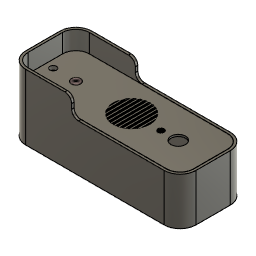
voipdoorbell-modeled (Autodesk Fusion 360 design; units mm, degrees)
Autodesk Fusion 360 part; units mm, degrees
sketch "Sketch1" plane through (0, 0, 0) normal (0, 1, 0) x (1, 0, 0)
  line L0 (-29, 11.5) -> (29, 11.5) construction
  line L1 (29, 11.5) -> (29, -11.5) construction
  line L2 (29, -11.5) -> (-29, -11.5) construction
  line L3 (-29, -11.5) -> (-29, 11.5) construction
  line L4 (-29, 11.5) -> (29, -11.5) construction
  line L5 (29, 11.5) -> (-29, -11.5) construction
  circle A0 centre (-29, 11.5) radius 1.25
  circle A1 centre (29, 11.5) radius 1.25
  circle A2 centre (29, -11.5) radius 1.25
  circle A3 centre (-29, -11.5) radius 1.25
  circle A4 centre (-29, 11.5) radius 2.75
  circle A5 centre (29, 11.5) radius 2.75
  circle A6 centre (29, -11.5) radius 2.75
  circle A7 centre (-29, -11.5) radius 2.75
  line L6 (56.5, 25) -> (-56.5, 25)
  line L7 (-67.5, 14) -> (-67.5, -14)
  line L8 (-56.5, -25) -> (56.5, -25)
  line L9 (67.5, -14) -> (67.5, 14)
  line L10 (67.5, 25) -> (-67.5, -25) construction
  line L11 (-67.5, 25) -> (67.5, -25) construction
  arc A8 (-67.5, -14) -> (-56.5, -25) centre (-56.5, -14) ccw
  arc A9 (-56.5, 25) -> (-67.5, 14) centre (-56.5, 14) ccw
  arc A10 (67.5, 14) -> (56.5, 25) centre (56.5, 14) ccw
  arc A11 (56.5, -25) -> (67.5, -14) centre (56.5, -14) ccw
  line L12 (69.5, -14) -> (69.5, 14)
  arc A12 (69.5, 14) -> (56.5, 27) centre (56.5, 14) ccw
  line L13 (56.5, 27) -> (-56.5, 27)
  arc A13 (-56.5, 27) -> (-69.5, 14) centre (-56.5, 14) ccw
  line L14 (-69.5, 14) -> (-69.5, -14)
  arc A14 (-69.5, -14) -> (-56.5, -27) centre (-56.5, -14) ccw
  line L15 (-56.5, -27) -> (56.5, -27)
  arc A15 (56.5, -27) -> (69.5, -14) centre (56.5, -14) ccw
  circle A16 centre (60, 0) radius 5
  circle A17 centre (56.5, -14) radius 1.5
  circle A18 centre (56.5, 14) radius 1.5
  circle A19 centre (-56.5, -14) radius 1.5
  circle A20 centre (-56.5, 14) radius 1.5
  dimension "d1" = 58
  dimension "d2" = 23
  dimension "d3" = 2.5
  dimension "d4" = 2.5
  dimension "d5" = 2.5
  dimension "d6" = 2.5
  dimension "d7" = 1.5
  dimension "d8" = 1.5
  dimension "d9" = 1.5
  dimension "d10" = 1.5
  dimension "d11" = 11
  dimension "d12" = 11
  dimension "d13" = 11
  dimension "d14" = 11
  dimension "d15" = 135
  dimension "d16" = 50
  dimension "d17" = 2
  dimension "d53" = 10
  dimension "d79" = 3
  dimension "d80" = 3
  dimension "d81" = 3
  dimension "d82" = 3
  constraint horizontal L0
  constraint perpendicular L0 L1
  constraint parallel L0 L2
  constraint parallel L1 L3
  constraint coincident L4 origin
  constraint coincident L5 origin
  constraint coincident L0.start L3.end
  constraint coincident L0.end L1.start
  constraint coincident L1.end L2.start
  constraint coincident L2.end L3.start
  constraint horizontal L6
  constraint perpendicular L6 L7
  constraint parallel L6 L8
  constraint parallel L7 L9
  constraint coincident L10 origin
  constraint coincident L11 origin
  constraint coincident L10.end L8
  constraint coincident L10.end L7
  constraint tangent L8 A8
  constraint tangent L7 A8
  constraint coincident L11.start L7
  constraint coincident L11.start L6
  constraint tangent L7 A9
  constraint tangent L6 A9
  constraint coincident L10.start L9
  constraint coincident L10.start L6
  constraint tangent L9 A10
  constraint tangent L6 A10
  constraint coincident L11.end L9
  constraint coincident L11.end L8
  constraint tangent L9 A11
  constraint tangent L8 A11
  constraint concentric A11 A17
  constraint concentric A10 A18
  constraint concentric A8 A19
  constraint concentric A9 A20
  measures "d1" distance of L0.start L0.end
  measures "d2" distance of L0.end L1.end
  measures "d3" diameter of A0
  measures "d4" diameter of A3
  measures "d5" diameter of A1
  measures "d6" diameter of A2
  measures "d11" radius of A8
  measures "d12" radius of A9
  measures "d13" radius of A10
  measures "d14" radius of A11
  measures "d15" distance of L7 L9
  measures "d16" distance of L6 L8
  measures "d53" diameter of A16
  measures "d79" diameter of A20
  measures "d80" diameter of A19
  measures "d81" diameter of A17
  measures "d82" diameter of A18
other "Base Mesh Feature1"
other "Base Mesh Feature2"
other "Modify1"
other "Modify2"
other "Modify3"
extrude "Extrude1" add sketch "Sketch1" against normal blind 2 contours A0 | A1 | A2 | A3 | A4 | A5 | A6 | A7 | L6 L7 L8 L9 A8 A9 A10 A11 | L12 A12 L13 A13 L14 A14 L15 A15 | A16 | A17 | A18 | A19 | A20 makes body 1
extrude "Extrude2" add sketch "Sketch1" along normal blind 2 contours A4 | A5 | A6 | A7 bodies 1
extrude "Extrude3" add sketch "Sketch1" along normal blind 35 contours L12 A12 L13 A13 L14 A14 L15 A15 bodies 1
sketch "Sketch2" plane through (0, 35, 0) normal (0, 1, 0) x (-1, 0, 0)
  arc A0 (-56.5, 25) -> (-67.5, 14) centre (-56.5, 14) ccw
  line L0 (-56.5, 25) -> (56.5, 25)
  arc A1 (67.5, 14) -> (56.5, 25) centre (56.5, 14) ccw
  line L1 (67.5, 14) -> (67.5, -14)
  arc A2 (56.5, -25) -> (67.5, -14) centre (56.5, -14) ccw
  line L2 (56.5, -25) -> (-56.5, -25)
  arc A3 (-67.5, -14) -> (-56.5, -25) centre (-56.5, -14) ccw
  line L3 (-67.5, -14) -> (-67.5, 14)
  arc A4 (-56.5, 27) -> (-69.5, 14) centre (-56.5, 14) ccw
  line L4 (-69.5, 14) -> (-69.5, -14)
  arc A5 (-69.5, -14) -> (-56.5, -27) centre (-56.5, -14) ccw
  line L5 (-56.5, -27) -> (56.5, -27)
  arc A6 (56.5, -27) -> (69.5, -14) centre (56.5, -14) ccw
  line L6 (69.5, -14) -> (69.5, 14)
  arc A7 (69.5, 14) -> (56.5, 27) centre (56.5, 14) ccw
  line L7 (56.5, 27) -> (-56.5, 27)
  line L8 (67.35, 14) -> (67.35, -14)
  arc A8 (56.5, -24.85) -> (67.35, -14) centre (56.5, -14) ccw
  line L9 (56.5, -24.85) -> (-56.5, -24.85)
  arc A9 (-67.35, -14) -> (-56.5, -24.85) centre (-56.5, -14) ccw
  line L10 (-67.35, -14) -> (-67.35, 14)
  arc A10 (-56.5, 24.85) -> (-67.35, 14) centre (-56.5, 14) ccw
  line L11 (-56.5, 24.85) -> (56.5, 24.85)
  arc A11 (67.35, 14) -> (56.5, 24.85) centre (56.5, 14) ccw
  circle A12 centre (42.5, 0) radius 3.75
  line L12 (54.25, 10.5) -> (42, 10.5) construction
  line L13 (42, 10.5) -> (42, -10.5) construction
  line L14 (42, -10.5) -> (54.25, -10.5) construction
  line L15 (54.25, -10.5) -> (54.25, 10.5) construction
  circle A13 centre (42, 10.5) radius 1
  circle A14 centre (42, -10.5) radius 1
  circle A15 centre (54.25, -10.5) radius 1
  circle A16 centre (54.25, 10.5) radius 1
  circle A17 centre (-41, 0) radius 6
  circle A18 centre (-27, 0) radius 2.5
  circle A19 centre (-3, 0) radius 15
  circle A20 centre (-3, 0) radius 18.5
  line L16 (-56.5, 23.3) -> (56.5, 23.3)
  arc A21 (65.8, 14) -> (56.5, 23.3) centre (56.5, 14) ccw
  line L17 (65.8, 14) -> (65.8, -14)
  arc A22 (56.5, -23.3) -> (65.8, -14) centre (56.5, -14) ccw
  line L18 (56.5, -23.3) -> (-56.5, -23.3)
  arc A23 (-65.8, -14) -> (-56.5, -23.3) centre (-56.5, -14) ccw
  line L19 (-65.8, -14) -> (-65.8, 14)
  arc A24 (-56.5, 23.3) -> (-65.8, 14) centre (-56.5, 14) ccw
  circle A25 centre (42, -10.5) radius 2
  circle A26 centre (54.25, -10.5) radius 2
  circle A27 centre (54.25, 10.5) radius 2
  circle A28 centre (42, 10.5) radius 2
  dimension "d24" = -0.15
  dimension "d25" = 7.5
  dimension "d26" = 25
  dimension "d27" = 25
  dimension "d28" = 2
  dimension "d29" = 2
  dimension "d30" = 2
  dimension "d31" = 2
  dimension "d32" = 21
  dimension "d33" = 12.25
  dimension "d34" = 10.5
  dimension "d35" = 0.5
  dimension "d37" = 12
  dimension "d39" = 30
  dimension "d40" = 37
  dimension "d41" = 5
  dimension "d42" = 1.7
  dimension "d126" = 4
  dimension "d127" = 4
  dimension "d128" = 4
  dimension "d129" = 4
  constraint horizontal L12
  constraint vertical L13
  constraint horizontal L14
  constraint vertical L15
  constraint coincident L12.end L13.start
  constraint coincident L13.end L14.start
  constraint coincident L14.end L15.start
  constraint coincident L12.start L15.end
  constraint concentric A19 A20
  constraint concentric A16 A27
  constraint concentric A13 A28
  measures "d25" diameter of A12
  measures "d26" distance of L1 A12.centre
  measures "d27" distance of L2 A12.centre
  measures "d28" diameter of A13
  measures "d29" diameter of A14
  measures "d30" diameter of A15
  measures "d31" diameter of A16
  measures "d32" distance of L12.end L13.end
  measures "d33" distance of L12.start L12.end
  measures "d34" distance of A12.centre L12
  measures "d35" distance of A12.centre L13
  measures "d37" diameter of A17
  measures "d39" diameter of A19
  measures "d40" diameter of A20
  measures "d41" diameter of A18
  measures "d126" diameter of A25
  measures "d127" diameter of A26
  measures "d128" diameter of A27
  measures "d129" diameter of A28
extrude "Extrude4" add sketch "Sketch2" against normal blind 24.95 separate body contours L8 A8 L9 A9 L10 A10 L11 A11 makes body 2
extrude "Extrude5" add sketch "Sketch2" along normal blind 1.5 contours L8 A8 L9 A9 L10 A10 L11 A11 | A13 | A14 | A15 | A16 | A20 | L16 A21 L17 A22 L18 A23 L19 A24 | A25 | A26 | A27 | A28 bodies 2
extrude "Extrude7" cut sketch "Sketch1" against normal blind 16 contours A16 bodies 1
extrude "Extrude8" add 1 faces at (18.8333, 35, 25.6667) along direction (0, 1, 0) blind 1.5 on bodies 1 bodies 1
sketch "Sketch4" plane through (0, 36.5, 0) normal (0, 1, 0) x (-1, 0, 0)
  arc A0 (-56.5, 25) -> (-67.5, 14) centre (-56.5, 14) ccw
  line L0 (-56.5, 25) -> (56.5, 25)
  arc A1 (67.5, 14) -> (56.5, 25) centre (56.5, 14) ccw
  line L1 (67.5, 14) -> (67.5, -14)
  arc A2 (56.5, -25) -> (67.5, -14) centre (56.5, -14) ccw
  line L2 (56.5, -25) -> (-56.5, -25)
  arc A3 (-67.5, -14) -> (-56.5, -25) centre (-56.5, -14) ccw
  line L3 (-67.5, -14) -> (-67.5, 14)
  arc A4 (-56.5, 27) -> (-69.5, 14) centre (-56.5, 14) ccw
  line L4 (-69.5, 14) -> (-69.5, -14)
  arc A5 (-69.5, -14) -> (-56.5, -27) centre (-56.5, -14) ccw
  line L5 (-56.5, -27) -> (56.5, -27)
  arc A6 (56.5, -27) -> (69.5, -14) centre (56.5, -14) ccw
  line L6 (69.5, -14) -> (69.5, 14)
  arc A7 (69.5, 14) -> (56.5, 27) centre (56.5, 14) ccw
  line L7 (56.5, 27) -> (-56.5, 27)
  line L8 (19, 39) -> (19, -40)
  constraint vertical L8
extrude "Extrude9" add sketch "Sketch4" along normal blind 15 contours L0 A1 L1 A2 L2 L5 A6 L6 A7 L7 L8 bodies 1
fillet "Fillet3" radius 5.5 2 edges at (-19, 51.5, -26) (-19, 51.5, 26) on bodies 1
fillet "Fillet4" radius 5.5 2 edges at (-19, 36.5, 26) (-19, 36.5, -26) on bodies 1
sketch "Sketch5" plane through (-67.35, 0, 0) normal (-1, 0, 0) x (0, 0, 1)
  line L0 (-14, 36.5) -> (-14, 10.05)
  line L1 (-14, 10.05) -> (14, 10.05)
  line L2 (14, 10.05) -> (14, 36.5)
  line L3 (14, 36.5) -> (-14, 36.5)
  line L4 (4.9486, 10.05) -> (-4.9486, 10.05)
  line L5 (-4.9486, 10.05) -> (-4.9486, 31.95)
  line L6 (-4.9486, 31.95) -> (4.9486, 31.95)
  line L7 (4.9486, 31.95) -> (4.9486, 10.05)
  line L8 (4.9486, 10.05) -> (-4.9486, 31.95) construction
  line L9 (-4.9486, 10.05) -> (4.9486, 31.95) construction
  point P0 (0, 21)
  constraint horizontal L4
  constraint perpendicular L4 L5
  constraint parallel L4 L6
  constraint parallel L5 L7
  constraint coincident L8 P0
  constraint coincident L9 P0
  constraint coincident L1 L4.start
extrude "Extrude10" cut sketch "Sketch5" against normal blind 5 contours L1 L4 L5 L6 L7 bodies 2
extrude "Extrude11" cut 1 faces at (-66.3167, 31.95, 1.6495) along direction (0, 1, 0) blind 3 on bodies 2 bodies 2
sketch "Sketch6" plane through (-67.5, 0, 0) normal (1, 0, 0) x (0, 0, -1)
  line L0 (-14, 0) -> (14, 0)
  line L1 (14, 0) -> (14, 51.5)
  line L2 (14, 51.5) -> (-14, 51.5)
  line L3 (-14, 51.5) -> (-14, 0)
  line L4 (4.2362, 7.1464) -> (-4.2553, 7.1464)
  line L5 (-4.2553, 7.1464) -> (-4.2553, 24.7678)
  line L6 (-4.2553, 24.7678) -> (4.2362, 24.7678)
  line L7 (4.2362, 24.7678) -> (4.2362, 7.1464)
  line L8 (4.2362, 7.1464) -> (-4.2553, 24.7678) construction
  line L9 (-4.2553, 7.1464) -> (4.2362, 24.7678) construction
  point P0 (-0.0095, 15.9571)
  constraint horizontal L4
  constraint perpendicular L4 L5
  constraint parallel L4 L6
  constraint parallel L5 L7
  constraint coincident L8 P0
  constraint coincident L9 P0
extrude "Extrude12" add sketch "Sketch6" along normal blind 4.5 separate body contours L4 L5 L6 L7 makes body 3
sketch "Sketch7" plane through (0, 7.1464, 0) normal (0, -1, 0) x (1, 0, 0)
  line L0 (-67.5, 4.2553) -> (-67.5, -4.2362)
  line L1 (-67.5, -4.2362) -> (-63, -4.2362)
  line L2 (-63, -4.2362) -> (-63, 4.2553)
  line L3 (-63, 4.2553) -> (-67.5, 4.2553)
  circle A0 centre (-49.4164, -0.0071) radius 1.25
  circle A1 centre (-49.4164, -0.0071) radius 1.5
  dimension "d70" = 2.5
  dimension "d132" = 3
  constraint concentric A0 A1
  measures "d70" diameter of A0
  measures "d132" diameter of A1
extrude "Extrude14" add 1 faces at (-63, 18.894, 1.4248) along direction (1, 0, 0) blind 0.5 on bodies 3 bodies 3
extrude "Extrude16" add 1 faces at (-67.5, 18.894, 1.4248) along direction (-1, 0, 0) blind 1 on bodies 3 bodies 3 1
extrude "Extrude17" cut sketch "Sketch1" against normal blind 11 contours A17 | A18 | A19 | A20 bodies 3
sketch "Sketch9" plane through (0, 36.5, 0) normal (0, 1, 0) x (-1, 0, 0)
  circle A0 centre (42.5, 0) radius 3.75
  circle A1 centre (-3, 0) radius 15
  circle A2 centre (-41, 0) radius 6
  circle A3 centre (-27, 0) radius 2.5
  arc A4 (56.5, -24.85) -> (67.35, -14) centre (56.5, -14) ccw
  line L0 (67.35, -14) -> (67.35, 14)
  arc A5 (67.35, 14) -> (56.5, 24.85) centre (56.5, 14) ccw
  line L1 (56.5, 24.85) -> (-56.5, 24.85)
  arc A6 (-56.5, 24.85) -> (-67.35, 14) centre (-56.5, 14) ccw
  line L2 (-67.35, 14) -> (-67.35, -14)
  arc A7 (-67.35, -14) -> (-56.5, -24.85) centre (-56.5, -14) ccw
  line L3 (-56.5, -24.85) -> (56.5, -24.85)
  line L4 (13, 20) -> (13, -20)
  line L5 (11.5, 20) -> (11.5, -20)
  line L6 (10, 20) -> (10, -20)
  line L7 (8.5, 20) -> (8.5, -20)
  line L8 (7, 20) -> (7, -20)
  line L9 (5.5, 20) -> (5.5, -20)
  line L10 (4, 20) -> (4, -20)
  line L11 (2.5, 20) -> (2.5, -20)
  line L12 (1, 20) -> (1, -20)
  line L13 (-0.5, 20) -> (-0.5, -20)
  line L14 (-2, 20) -> (-2, -20)
  line L15 (-3.5, 20) -> (-3.5, -20)
  line L16 (-5, 20) -> (-5, -20)
  line L17 (-6.5, 20) -> (-6.5, -20)
  line L18 (-8, 20) -> (-8, -20)
  line L19 (-9.5, 20) -> (-9.5, -20)
  line L20 (-11, 20) -> (-11, -20)
  line L21 (-12.5, 20) -> (-12.5, -20)
  line L22 (-14, 20) -> (-14, -20)
  line L23 (-15.5, 20) -> (-15.5, -20)
  line L24 (-17, 20) -> (-17, -20)
  line L25 (-18.5, 20) -> (-18.5, -20)
  line L26 (-24.757, 5.9816) -> (-24.757, -6.5184)
  line L27 (-25.257, 5.9816) -> (-25.257, -6.5184)
  line L28 (-25.757, 5.9816) -> (-25.757, -6.5184)
  line L29 (-26.257, 5.9816) -> (-26.257, -6.5184)
  line L30 (-26.757, 5.9816) -> (-26.757, -6.5184)
  line L31 (-27.257, 5.9816) -> (-27.257, -6.5184)
  line L32 (-27.757, 5.9816) -> (-27.757, -6.5184)
  line L33 (-28.257, 5.9816) -> (-28.257, -6.5184)
  line L34 (-28.757, 5.9816) -> (-28.757, -6.5184)
  line L35 (-29.257, 5.9816) -> (-29.257, -6.5184)
  line L36 (-29.757, 5.9816) -> (-29.757, -6.5184)
  dimension "d85" = 1.5
  dimension "d86" = 3
  dimension "d87" = 4.5
  dimension "d88" = 6
  dimension "d89" = 7.5
  dimension "d90" = 9
  dimension "d91" = 10.5
  dimension "d92" = 12
  dimension "d93" = 13.5
  dimension "d94" = 15
  dimension "d95" = 16.5
  dimension "d96" = 18
  dimension "d97" = 19.5
  dimension "d98" = 21
  dimension "d99" = 22.5
  dimension "d100" = 24
  dimension "d101" = 25.5
  dimension "d102" = 27
  dimension "d103" = 28.5
  dimension "d104" = 30
  dimension "d105" = 31.5
  dimension "d114" = 0.5
  dimension "d115" = 1
  dimension "d116" = 1.5
  dimension "d117" = 2
  dimension "d118" = 2.5
  dimension "d119" = 3
  dimension "d120" = 3.5
  dimension "d121" = 4
  dimension "d122" = 4.5
  dimension "d123" = 5
  constraint perpendicular L3 L4
  constraint vertical L26
extrude "Extrude18" add sketch "Sketch9" against normal blind 1.5 contours A1 L5 | A1 L5 L6 | A1 L6 L7 | A1 L7 L8 | A1 L8 L9 | A1 L9 L10 | A1 L10 L11 | A1 L11 L12 | A1 L12 L13 | A1 L13 L14 | A1 L14 L15 | A1 L15 L16 | A1 L16 L17 | A1 L17 L18 | A1 L18 L19 | A1 L19 L20 | A1 L20 L21 | A1 L21 L22 | A1 L22 L23 | A1 L23 L24 | A1 L24 bodies 2
extrude "Extrude19" cut sketch "Sketch9" against normal blind 5 contours A1 L5 L6 | A1 L7 L8 | A1 L9 L10 | A1 L11 L12 | A1 L13 L14 | A1 L15 L16 | A1 L17 L18 | A1 L19 L20 | A1 L21 L22 | A1 L23 L24 bodies 2
extrude "Extrude20" cut sketch "Sketch9" against normal blind 1 contours A1 L5 | A1 L6 L7 | A1 L8 L9 | A1 L10 L11 | A1 L12 L13 | A1 L14 L15 | A1 L16 L17 | A1 L18 L19 | A1 L20 L21 | A1 L22 L23 | A1 L24 bodies 2
extrude "Extrude21" add sketch "Sketch9" against normal blind 0.5 contours A1 L5 L6 | A1 L7 L8 | A1 L9 L10 | A1 L11 L12 | A1 L13 L14 | A1 L15 L16 | A1 L17 L18 | A1 L19 L20 | A1 L21 L22 | A1 L23 L24 bodies 2
extrude "Extrude22" add sketch "Sketch9" against normal blind 1 contours A3 L26 L27 | A3 L28 L29 | A3 L30 L31 | A3 L32 L33 | A3 L34 L35 bodies 2
extrude "Extrude23" add sketch "Sketch2" against normal blind 3.3 contours A25 | A26 | A27 | A28 bodies 2
sketch "Sketch10" plane through (0, 36.5, 0) normal (0, 1, 0) x (-1, 0, 0)
  arc A0 (-29.257, 1.0752) -> (-29.257, -1.0752) centre (-27, 0) ccw
  line L0 (-29.257, 1.0752) -> (-29.257, -1.0752)
  arc A1 (-25.757, -2.1691) -> (-25.257, -1.7922) centre (-27, 0) ccw
  line L1 (-25.757, -2.1691) -> (-25.757, 2.1691)
  arc A2 (-25.257, 1.7922) -> (-25.757, 2.1691) centre (-27, 0) ccw
  line L2 (-25.257, 1.7922) -> (-25.257, -1.7922)
  line L3 (-28.757, -1.7785) -> (-28.757, 1.7785)
  arc A3 (-28.257, 2.161) -> (-28.757, 1.7785) centre (-27, 0) ccw
  line L4 (-28.257, 2.161) -> (-28.257, -2.161)
  arc A4 (-28.757, -1.7785) -> (-28.257, -2.161) centre (-27, 0) ccw
  arc A5 (-26.757, -2.4882) -> (-26.257, -2.387) centre (-27, 0) ccw
  line L5 (-26.757, -2.4882) -> (-26.757, 2.4882)
  arc A6 (-26.257, 2.387) -> (-26.757, 2.4882) centre (-27, 0) ccw
  line L6 (-26.257, 2.387) -> (-26.257, -2.387)
  line L7 (-27.757, -2.3826) -> (-27.757, 2.3826)
  arc A7 (-27.257, 2.4868) -> (-27.757, 2.3826) centre (-27, 0) ccw
  line L8 (-27.257, 2.4868) -> (-27.257, -2.4868)
  arc A8 (-27.757, -2.3826) -> (-27.257, -2.4868) centre (-27, 0) ccw
  arc A9 (-17, 5.3852) -> (-17, -5.3852) centre (-3, 0) ccw
  line L9 (-17, 5.3852) -> (-17, -5.3852)
  arc A10 (-6.5, -14.586) -> (-5, -14.8661) centre (-3, 0) ccw
  line L10 (-6.5, -14.586) -> (-6.5, 14.586)
  arc A11 (-5, 14.8661) -> (-6.5, 14.586) centre (-3, 0) ccw
  line L11 (-5, 14.8661) -> (-5, -14.8661)
  arc A12 (5.5, -12.3592) -> (7, -11.1803) centre (-3, 0) ccw
  line L12 (5.5, -12.3592) -> (5.5, 12.3592)
  arc A13 (7, 11.1803) -> (5.5, 12.3592) centre (-3, 0) ccw
  line L13 (7, 11.1803) -> (7, -11.1803)
  arc A14 (2.5, -13.9553) -> (4, -13.2665) centre (-3, 0) ccw
  line L14 (2.5, -13.9553) -> (2.5, 13.9553)
  arc A15 (4, 13.2665) -> (2.5, 13.9553) centre (-3, 0) ccw
  line L15 (4, 13.2665) -> (4, -13.2665)
  arc A16 (-9.5, -13.5185) -> (-8, -14.1421) centre (-3, 0) ccw
  line L16 (-9.5, -13.5185) -> (-9.5, 13.5185)
  arc A17 (-8, 14.1421) -> (-9.5, 13.5185) centre (-3, 0) ccw
  line L17 (-8, 14.1421) -> (-8, -14.1421)
  line L18 (-15.5, -8.2916) -> (-15.5, 8.2916)
  arc A18 (-14, 10.198) -> (-15.5, 8.2916) centre (-3, 0) ccw
  line L19 (-14, 10.198) -> (-14, -10.198)
  arc A19 (-15.5, -8.2916) -> (-14, -10.198) centre (-3, 0) ccw
  line L20 (-3.5, -14.9917) -> (-3.5, 14.9917)
  arc A20 (-2, 14.9666) -> (-3.5, 14.9917) centre (-3, 0) ccw
  line L21 (-2, 14.9666) -> (-2, -14.9666)
  arc A21 (-3.5, -14.9917) -> (-2, -14.9666) centre (-3, 0) ccw
  line L22 (8.5, -9.6307) -> (8.5, 9.6307)
  arc A22 (10, 7.4833) -> (8.5, 9.6307) centre (-3, 0) ccw
  line L23 (10, 7.4833) -> (10, -7.4833)
  arc A23 (8.5, -9.6307) -> (10, -7.4833) centre (-3, 0) ccw
  line L24 (-0.5, -14.7902) -> (-0.5, 14.7902)
  arc A24 (1, 14.4568) -> (-0.5, 14.7902) centre (-3, 0) ccw
  line L25 (1, 14.4568) -> (1, -14.4568)
  arc A25 (-0.5, -14.7902) -> (1, -14.4568) centre (-3, 0) ccw
  line L26 (-12.5, -11.6082) -> (-12.5, 11.6082)
  arc A26 (-11, 12.6886) -> (-12.5, 11.6082) centre (-3, 0) ccw
  line L27 (-11, 12.6886) -> (-11, -12.6886)
  arc A27 (-12.5, -11.6082) -> (-11, -12.6886) centre (-3, 0) ccw
  line L28 (11.5, -3.8406) -> (11.5, 3.8406)
  arc A28 (11.5, -3.8406) -> (11.5, 3.8406) centre (-3, 0) ccw
  line L29 (-24.757, -1.1041) -> (-24.757, 1.1041)
  arc A29 (-24.757, -1.1041) -> (-24.757, 1.1041) centre (-27, 0) ccw
  circle A30 centre (-41, 0) radius 6
  circle A31 centre (42.5, 0) radius 3.75
  arc A32 (56.5, -24.85) -> (67.35, -14) centre (56.5, -14) ccw
  line L30 (67.35, -14) -> (67.35, 14)
  arc A33 (67.35, 14) -> (56.5, 24.85) centre (56.5, 14) ccw
  line L31 (56.5, 24.85) -> (-56.5, 24.85)
  arc A34 (-56.5, 24.85) -> (-67.35, 14) centre (-56.5, 14) ccw
  line L32 (-67.35, 14) -> (-67.35, -14)
  arc A35 (-67.35, -14) -> (-56.5, -24.85) centre (-56.5, -14) ccw
  line L33 (-56.5, -24.85) -> (56.5, -24.85)
  circle A36 centre (59, 0) radius 2.75
  circle A37 centre (59, 0) radius 3.75
  line L34 (46.5, 3.5) -> (46.5, -3.3735)
  dimension "d135" = 5.5
  dimension "d148" = 1
  constraint vertical L34
  measures "d135" diameter of A36
extrude "Extrude25" cut sketch "Sketch10" against normal blind 4 contours A36 bodies 2
extrude "Extrude26" add sketch "Sketch10" against normal blind 4 contours A36 bodies 2
extrude "Extrude27" cut sketch "Sketch10" against normal blind 3.1 contours A36 bodies 2 makes body 4 at (-59.8259, 33.4, -0.3977)
extrude "Extrude28" add sketch "Sketch10" against normal blind 4 contours A37 bodies 2 4
extrude "Extrude30" cut 1 faces at (-64.1667, 24.7678, 1.4248) along direction (0, -1, 0) blind 2.5 on bodies 3 bodies 3
extrude "Extrude31" cut sketch "Sketch10" against normal blind 6 contours A36 | A37 bodies 2
extrude "Extrude32" add sketch "Sketch10" against normal blind 1.5 contours A36 | A37 bodies 2
sketch "Sketch11" plane through (0, 36.5, 0) normal (0, 1, 0) x (-1, 0, 0)
  line L0 (67.35, -14) -> (67.35, 14)
  arc A0 (67.35, 14) -> (56.5, 24.85) centre (56.5, 14) ccw
  line L1 (56.5, 24.85) -> (-56.5, 24.85)
  arc A1 (-56.5, 24.85) -> (-67.35, 14) centre (-56.5, 14) ccw
  line L2 (-67.35, 14) -> (-67.35, -14)
  arc A2 (-67.35, -14) -> (-56.5, -24.85) centre (-56.5, -14) ccw
  line L3 (-56.5, -24.85) -> (56.5, -24.85)
  arc A3 (56.5, -24.85) -> (67.35, -14) centre (56.5, -14) ccw
  circle A4 centre (-41, 0) radius 6
  line L4 (-24.757, -1.1041) -> (-24.757, 1.1041)
  arc A5 (-24.757, -1.1041) -> (-24.757, 1.1041) centre (-27, 0) ccw
  line L5 (11.5, -3.8406) -> (11.5, 3.8406)
  arc A6 (11.5, -3.8406) -> (11.5, 3.8406) centre (-3, 0) ccw
  line L6 (-12.5, -11.6082) -> (-12.5, 11.6082)
  arc A7 (-11, 12.6886) -> (-12.5, 11.6082) centre (-3, 0) ccw
  line L7 (-11, 12.6886) -> (-11, -12.6886)
  arc A8 (-12.5, -11.6082) -> (-11, -12.6886) centre (-3, 0) ccw
  line L8 (-0.5, -14.7902) -> (-0.5, 14.7902)
  arc A9 (1, 14.4568) -> (-0.5, 14.7902) centre (-3, 0) ccw
  line L9 (1, 14.4568) -> (1, -14.4568)
  arc A10 (-0.5, -14.7902) -> (1, -14.4568) centre (-3, 0) ccw
  line L10 (8.5, -9.6307) -> (8.5, 9.6307)
  arc A11 (10, 7.4833) -> (8.5, 9.6307) centre (-3, 0) ccw
  line L11 (10, 7.4833) -> (10, -7.4833)
  arc A12 (8.5, -9.6307) -> (10, -7.4833) centre (-3, 0) ccw
  line L12 (-3.5, -14.9917) -> (-3.5, 14.9917)
  arc A13 (-2, 14.9666) -> (-3.5, 14.9917) centre (-3, 0) ccw
  line L13 (-2, 14.9666) -> (-2, -14.9666)
  arc A14 (-3.5, -14.9917) -> (-2, -14.9666) centre (-3, 0) ccw
  line L14 (-15.5, -8.2916) -> (-15.5, 8.2916)
  arc A15 (-14, 10.198) -> (-15.5, 8.2916) centre (-3, 0) ccw
  line L15 (-14, 10.198) -> (-14, -10.198)
  arc A16 (-15.5, -8.2916) -> (-14, -10.198) centre (-3, 0) ccw
  arc A17 (-9.5, -13.5185) -> (-8, -14.1421) centre (-3, 0) ccw
  line L16 (-9.5, -13.5185) -> (-9.5, 13.5185)
  arc A18 (-8, 14.1421) -> (-9.5, 13.5185) centre (-3, 0) ccw
  line L17 (-8, 14.1421) -> (-8, -14.1421)
  arc A19 (2.5, -13.9553) -> (4, -13.2665) centre (-3, 0) ccw
  line L18 (2.5, -13.9553) -> (2.5, 13.9553)
  arc A20 (4, 13.2665) -> (2.5, 13.9553) centre (-3, 0) ccw
  line L19 (4, 13.2665) -> (4, -13.2665)
  arc A21 (5.5, -12.3592) -> (7, -11.1803) centre (-3, 0) ccw
  line L20 (5.5, -12.3592) -> (5.5, 12.3592)
  arc A22 (7, 11.1803) -> (5.5, 12.3592) centre (-3, 0) ccw
  line L21 (7, 11.1803) -> (7, -11.1803)
  arc A23 (-6.5, -14.586) -> (-5, -14.8661) centre (-3, 0) ccw
  line L22 (-6.5, -14.586) -> (-6.5, 14.586)
  arc A24 (-5, 14.8661) -> (-6.5, 14.586) centre (-3, 0) ccw
  line L23 (-5, 14.8661) -> (-5, -14.8661)
  arc A25 (-17, 5.3852) -> (-17, -5.3852) centre (-3, 0) ccw
  line L24 (-17, 5.3852) -> (-17, -5.3852)
  line L25 (-27.757, -2.3826) -> (-27.757, 2.3826)
  arc A26 (-27.257, 2.4868) -> (-27.757, 2.3826) centre (-27, 0) ccw
  line L26 (-27.257, 2.4868) -> (-27.257, -2.4868)
  arc A27 (-27.757, -2.3826) -> (-27.257, -2.4868) centre (-27, 0) ccw
  arc A28 (-26.757, -2.4882) -> (-26.257, -2.387) centre (-27, 0) ccw
  line L27 (-26.757, -2.4882) -> (-26.757, 2.4882)
  arc A29 (-26.257, 2.387) -> (-26.757, 2.4882) centre (-27, 0) ccw
  line L28 (-26.257, 2.387) -> (-26.257, -2.387)
  line L29 (-28.757, -1.7785) -> (-28.757, 1.7785)
  arc A30 (-28.257, 2.161) -> (-28.757, 1.7785) centre (-27, 0) ccw
  line L30 (-28.257, 2.161) -> (-28.257, -2.161)
  arc A31 (-28.757, -1.7785) -> (-28.257, -2.161) centre (-27, 0) ccw
  arc A32 (-25.757, -2.1691) -> (-25.257, -1.7922) centre (-27, 0) ccw
  line L31 (-25.757, -2.1691) -> (-25.757, 2.1691)
  arc A33 (-25.257, 1.7922) -> (-25.757, 2.1691) centre (-27, 0) ccw
  line L32 (-25.257, 1.7922) -> (-25.257, -1.7922)
  arc A34 (-29.257, 1.0752) -> (-29.257, -1.0752) centre (-27, 0) ccw
  line L33 (-29.257, 1.0752) -> (-29.257, -1.0752)
  circle A35 centre (49.4164, -0.0071) radius 1.4415
  circle A36 centre (49.4164, -0.0071) radius 1.3693
  circle A37 centre (49.4164, -0.0071) radius 1.3125
  circle A38 centre (42.5, 0) radius 3.75
  constraint concentric A35 A36
  constraint concentric A35 A37
extrude "Extrude37" add 5 faces at (28.9237, 35.5, 0.3584) (27.9237, 35.5, 0.7203) (26.9792, 35.5, -0.8328) (26.0311, 35.5, 0.7957) (24.9237, 35.5, 0.5974) along direction (0, -1, 0) blind 0.5 on bodies 2 bodies 2
other "Modify4"
other "Modify5"
other "Modify6"
other "Modify7"
extrude "Extrude38" add 1 faces at (-18.8333, 10.05, -24.3333) along direction (0, -1, 0) blind 10 on bodies 2 bodies 2
extrude "Extrude39" add 1 faces at (-62.5, 17.2274, 1.4248) along direction (1, 0, 0) blind 4 on bodies 3 bodies 3
extrude "Extrude40" add 1 faces at (-61.5, 7.1464, 1.4248) along direction (0, -1, 0) blind 8 on bodies 3 bodies 3
extrude "Extrude41" add 1 faces at (-64.5, 22.2678, 1.4248) along direction (0, 1, 0) blind 12 on bodies 3 bodies 3
extrude "Extrude42" cut 1 faces at (-64.5, 34.2678, 1.4248) along direction (0, -1, 0) blind 2 on bodies 3 bodies 3
sketch "Sketch12" plane through (0, 32.2678, 0) normal (0, 1, 0) x (-1, 0, 0)
  line L0 (67.5, -4.2362) -> (67.5, 4.2553)
  line L1 (67.5, 4.2553) -> (58.5, 4.2553)
  line L2 (58.5, 4.2553) -> (58.5, -4.2362)
  line L3 (58.5, -4.2362) -> (67.5, -4.2362)
  circle A0 centre (61, 0) radius 1.45
  dimension "d191" = 2.9
  measures "d191" diameter of A0
extrude "Extrude43" cut sketch "Sketch12" against normal blind 24 contours A0 bodies 3
extrude "Extrude44" cut sketch "Sketch12" along normal blind 8 contours A0 bodies 2
sketch "Sketch13" plane through (0, 35, 0) normal (0, -1, 0) x (1, 0, 0)
  circle A0 centre (-61, 0) radius 1.45
  arc A1 (24.757, 1.1041) -> (24.757, -1.1041) centre (27, 0) ccw
  line L0 (24.757, 1.1041) -> (24.757, -1.1041)
  arc A2 (26.257, -2.387) -> (26.757, -2.4882) centre (27, 0) ccw
  line L1 (26.257, -2.387) -> (26.257, 2.387)
  arc A3 (26.757, 2.4882) -> (26.257, 2.387) centre (27, 0) ccw
  line L2 (26.757, 2.4882) -> (26.757, -2.4882)
  arc A4 (28.257, -2.161) -> (28.757, -1.7785) centre (27, 0) ccw
  line L3 (28.257, -2.161) -> (28.257, 2.161)
  arc A5 (28.757, 1.7785) -> (28.257, 2.161) centre (27, 0) ccw
  line L4 (28.757, 1.7785) -> (28.757, -1.7785)
  line L5 (27.257, -2.4868) -> (27.257, 2.4868)
  arc A6 (27.757, 2.3826) -> (27.257, 2.4868) centre (27, 0) ccw
  line L6 (27.757, 2.3826) -> (27.757, -2.3826)
  arc A7 (27.257, -2.4868) -> (27.757, -2.3826) centre (27, 0) ccw
  line L7 (25.257, -1.7922) -> (25.257, 1.7922)
  arc A8 (25.757, 2.1691) -> (25.257, 1.7922) centre (27, 0) ccw
  line L8 (25.757, 2.1691) -> (25.757, -2.1691)
  arc A9 (25.257, -1.7922) -> (25.757, -2.1691) centre (27, 0) ccw
  circle A10 centre (-42, -10.5) radius 2
  circle A11 centre (-54.25, -10.5) radius 2
  line L9 (11, 12.6886) -> (11, -12.6886)
  arc A12 (9.5, -13.5185) -> (11, -12.6886) centre (3, 0) ccw
  line L10 (9.5, -13.5185) -> (9.5, 13.5185)
  arc A13 (11, 12.6886) -> (9.5, 13.5185) centre (3, 0) ccw
  line L11 (-1, 14.4568) -> (-1, -14.4568)
  arc A14 (-2.5, -13.9553) -> (-1, -14.4568) centre (3, 0) ccw
  line L12 (-2.5, -13.9553) -> (-2.5, 13.9553)
  arc A15 (-1, 14.4568) -> (-2.5, 13.9553) centre (3, 0) ccw
  line L13 (-10, 7.4833) -> (-10, -7.4833)
  arc A16 (-11.5, -3.8406) -> (-10, -7.4833) centre (3, 0) ccw
  line L14 (-11.5, -3.8406) -> (-11.5, 3.8406)
  arc A17 (-10, 7.4833) -> (-11.5, 3.8406) centre (3, 0) ccw
  line L15 (2, 14.9666) -> (2, -14.9666)
  arc A18 (0.5, -14.7902) -> (2, -14.9666) centre (3, 0) ccw
  line L16 (0.5, -14.7902) -> (0.5, 14.7902)
  arc A19 (2, 14.9666) -> (0.5, 14.7902) centre (3, 0) ccw
  line L17 (14, 10.198) -> (14, -10.198)
  arc A20 (12.5, -11.6082) -> (14, -10.198) centre (3, 0) ccw
  line L18 (12.5, -11.6082) -> (12.5, 11.6082)
  arc A21 (14, 10.198) -> (12.5, 11.6082) centre (3, 0) ccw
  line L19 (8, 14.1421) -> (8, -14.1421)
  arc A22 (6.5, -14.586) -> (8, -14.1421) centre (3, 0) ccw
  line L20 (6.5, -14.586) -> (6.5, 14.586)
  arc A23 (8, 14.1421) -> (6.5, 14.586) centre (3, 0) ccw
  line L21 (-4, 13.2665) -> (-4, -13.2665)
  arc A24 (-5.5, -12.3592) -> (-4, -13.2665) centre (3, 0) ccw
  line L22 (-5.5, -12.3592) -> (-5.5, 12.3592)
  arc A25 (-4, 13.2665) -> (-5.5, 12.3592) centre (3, 0) ccw
  line L23 (-7, 11.1803) -> (-7, -11.1803)
  arc A26 (-8.5, -9.6307) -> (-7, -11.1803) centre (3, 0) ccw
  line L24 (-8.5, -9.6307) -> (-8.5, 9.6307)
  arc A27 (-7, 11.1803) -> (-8.5, 9.6307) centre (3, 0) ccw
  line L25 (5, 14.8661) -> (5, -14.8661)
  arc A28 (3.5, -14.9917) -> (5, -14.8661) centre (3, 0) ccw
  line L26 (3.5, -14.9917) -> (3.5, 14.9917)
  arc A29 (5, 14.8661) -> (3.5, 14.9917) centre (3, 0) ccw
  line L27 (17, 5.3852) -> (17, -5.3852)
  arc A30 (15.5, -8.2916) -> (17, -5.3852) centre (3, 0) ccw
  line L28 (15.5, -8.2916) -> (15.5, 8.2916)
  arc A31 (17, 5.3852) -> (15.5, 8.2916) centre (3, 0) ccw
  circle A32 centre (-42.5, 0) radius 3.75
  line L29 (29.257, -1.0752) -> (29.257, 1.0752)
  arc A33 (29.257, -1.0752) -> (29.257, 1.0752) centre (27, 0) ccw
  circle A34 centre (41, 0) radius 6
  line L30 (-65.8, 14) -> (-65.8, -14)
  arc A35 (-65.8, -14) -> (-56.5, -23.3) centre (-56.5, -14) ccw
  line L31 (-56.5, -23.3) -> (56.5, -23.3)
  arc A36 (56.5, -23.3) -> (65.8, -14) centre (56.5, -14) ccw
  line L32 (65.8, -14) -> (65.8, 14)
  arc A37 (65.8, 14) -> (56.5, 23.3) centre (56.5, 14) ccw
  line L33 (56.5, 23.3) -> (-56.5, 23.3)
  arc A38 (-56.5, 23.3) -> (-65.8, 14) centre (-56.5, 14) ccw
  circle A39 centre (-42, 10.5) radius 2
  circle A40 centre (-54.25, 10.5) radius 2
  circle A41 centre (-61, 0) radius 4.5
  dimension "d196" = 9
  constraint concentric A0 A41
  measures "d196" diameter of A41
extrude "Extrude45" add sketch "Sketch13" along normal blind 2.5 contours A41 bodies 2
sketch "Sketch14" plane through (0, 36.5, 0) normal (0, 1, 0) x (-1, 0, 0)
  circle A0 centre (61, 0) radius 1.45
  arc A1 (-29.257, 1.0752) -> (-29.257, -1.0752) centre (-27, 0) ccw
  line L0 (-29.257, 1.0752) -> (-29.257, -1.0752)
  arc A2 (-25.757, -2.1691) -> (-25.257, -1.7922) centre (-27, 0) ccw
  line L1 (-25.757, -2.1691) -> (-25.757, 2.1691)
  arc A3 (-25.257, 1.7922) -> (-25.757, 2.1691) centre (-27, 0) ccw
  line L2 (-25.257, 1.7922) -> (-25.257, -1.7922)
  line L3 (-28.757, -1.7785) -> (-28.757, 1.7785)
  arc A4 (-28.257, 2.161) -> (-28.757, 1.7785) centre (-27, 0) ccw
  line L4 (-28.257, 2.161) -> (-28.257, -2.161)
  arc A5 (-28.757, -1.7785) -> (-28.257, -2.161) centre (-27, 0) ccw
  arc A6 (-26.757, -2.4882) -> (-26.257, -2.387) centre (-27, 0) ccw
  line L5 (-26.757, -2.4882) -> (-26.757, 2.4882)
  arc A7 (-26.257, 2.387) -> (-26.757, 2.4882) centre (-27, 0) ccw
  line L6 (-26.257, 2.387) -> (-26.257, -2.387)
  line L7 (-27.757, -2.3826) -> (-27.757, 2.3826)
  arc A8 (-27.257, 2.4868) -> (-27.757, 2.3826) centre (-27, 0) ccw
  line L8 (-27.257, 2.4868) -> (-27.257, -2.4868)
  arc A9 (-27.757, -2.3826) -> (-27.257, -2.4868) centre (-27, 0) ccw
  arc A10 (-17, 5.3852) -> (-17, -5.3852) centre (-3, 0) ccw
  line L9 (-17, 5.3852) -> (-17, -5.3852)
  arc A11 (-6.5, -14.586) -> (-5, -14.8661) centre (-3, 0) ccw
  line L10 (-6.5, -14.586) -> (-6.5, 14.586)
  arc A12 (-5, 14.8661) -> (-6.5, 14.586) centre (-3, 0) ccw
  line L11 (-5, 14.8661) -> (-5, -14.8661)
  arc A13 (5.5, -12.3592) -> (7, -11.1803) centre (-3, 0) ccw
  line L12 (5.5, -12.3592) -> (5.5, 12.3592)
  arc A14 (7, 11.1803) -> (5.5, 12.3592) centre (-3, 0) ccw
  line L13 (7, 11.1803) -> (7, -11.1803)
  arc A15 (2.5, -13.9553) -> (4, -13.2665) centre (-3, 0) ccw
  line L14 (2.5, -13.9553) -> (2.5, 13.9553)
  arc A16 (4, 13.2665) -> (2.5, 13.9553) centre (-3, 0) ccw
  line L15 (4, 13.2665) -> (4, -13.2665)
  arc A17 (-9.5, -13.5185) -> (-8, -14.1421) centre (-3, 0) ccw
  line L16 (-9.5, -13.5185) -> (-9.5, 13.5185)
  arc A18 (-8, 14.1421) -> (-9.5, 13.5185) centre (-3, 0) ccw
  line L17 (-8, 14.1421) -> (-8, -14.1421)
  line L18 (-15.5, -8.2916) -> (-15.5, 8.2916)
  arc A19 (-14, 10.198) -> (-15.5, 8.2916) centre (-3, 0) ccw
  line L19 (-14, 10.198) -> (-14, -10.198)
  arc A20 (-15.5, -8.2916) -> (-14, -10.198) centre (-3, 0) ccw
  line L20 (-3.5, -14.9917) -> (-3.5, 14.9917)
  arc A21 (-2, 14.9666) -> (-3.5, 14.9917) centre (-3, 0) ccw
  line L21 (-2, 14.9666) -> (-2, -14.9666)
  arc A22 (-3.5, -14.9917) -> (-2, -14.9666) centre (-3, 0) ccw
  line L22 (8.5, -9.6307) -> (8.5, 9.6307)
  arc A23 (10, 7.4833) -> (8.5, 9.6307) centre (-3, 0) ccw
  line L23 (10, 7.4833) -> (10, -7.4833)
  arc A24 (8.5, -9.6307) -> (10, -7.4833) centre (-3, 0) ccw
  line L24 (-0.5, -14.7902) -> (-0.5, 14.7902)
  arc A25 (1, 14.4568) -> (-0.5, 14.7902) centre (-3, 0) ccw
  line L25 (1, 14.4568) -> (1, -14.4568)
  arc A26 (-0.5, -14.7902) -> (1, -14.4568) centre (-3, 0) ccw
  line L26 (-12.5, -11.6082) -> (-12.5, 11.6082)
  arc A27 (-11, 12.6886) -> (-12.5, 11.6082) centre (-3, 0) ccw
  line L27 (-11, 12.6886) -> (-11, -12.6886)
  arc A28 (-12.5, -11.6082) -> (-11, -12.6886) centre (-3, 0) ccw
  line L28 (11.5, -3.8406) -> (11.5, 3.8406)
  arc A29 (11.5, -3.8406) -> (11.5, 3.8406) centre (-3, 0) ccw
  circle A30 centre (-41, 0) radius 6
  line L29 (-24.757, -1.1041) -> (-24.757, 1.1041)
  arc A31 (-24.757, -1.1041) -> (-24.757, 1.1041) centre (-27, 0) ccw
  circle A32 centre (42.5, 0) radius 3.75
  arc A33 (56.5, -24.85) -> (67.35, -14) centre (56.5, -14) ccw
  line L30 (67.35, -14) -> (67.35, 14)
  arc A34 (67.35, 14) -> (56.5, 24.85) centre (56.5, 14) ccw
  line L31 (56.5, 24.85) -> (-56.5, 24.85)
  arc A35 (-56.5, 24.85) -> (-67.35, 14) centre (-56.5, 14) ccw
  line L32 (-67.35, 14) -> (-67.35, -14)
  arc A36 (-67.35, -14) -> (-56.5, -24.85) centre (-56.5, -14) ccw
  line L33 (-56.5, -24.85) -> (56.5, -24.85)
  circle A37 centre (61, 0) radius 2.7
  circle A38 centre (61, 0) radius 1.65
  dimension "d199" = 5.4
  dimension "d200" = 0.2
  constraint concentric A0 A37
  measures "d199" diameter of A37
extrude "Extrude46" cut sketch "Sketch14" against normal blind 4.6 contours A38 bodies 2
extrude "Extrude47" cut sketch "Sketch14" against normal blind 3.2 contours A37 bodies 2
